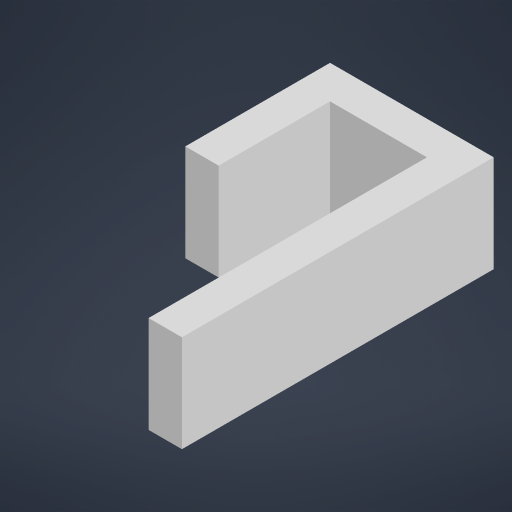
# Autodesk Inventor part: Hook_TestFit
Saved by Autodesk Inventor 2024 (Build 280153000, 153)
## iProperties
Created: 2023-07-11
Part Number: Hook_TestFit
Material: Generic
Document SubType Name: Modeling
Designer: User
Density: 1 g/cm^3
Appearance: Default
Author: User
Autodesk Inventor part; units mm, degrees
ref_plane "YZ Plane" through (0, 0, 0) normal (1, 0, 0) x (0, 1, 0)
ref_plane "XZ Plane" through (0, 0, 0) normal (0, 1, 0) x (-1, 0, 0)
ref_plane "XY Plane" through (0, 0, 0) normal (0, 0, 1) x (1, 0, 0)
sketch "Sketch1" plane through (0, 0, 0) normal (0, 0, 1) x (1, 0, 0)
  line L0 (0, 0) -> (-8.7, 0)
  line L1 (-8.7, 0) -> (-8.7, 8.7)
  line L2 (-8.7, 8.7) -> (0, 8.7)
  line L3 (0, 8.7) -> (0, 0)
  dimension "d0" = 8.7
  dimension "d1" = 8.7
  constraints: 8 end point, 2 parallel, 1 horizontal, 1 perpendicular
  measures "d0" distance of L1.end L2.end
  measures "d1" distance of L0.end L1.end
extrude "Extrusion1" add sketch "Sketch1" along normal blind 3
sketch "Sketch2" plane through (-8.7, 0, 0) normal (-1, 0, 0) x (0, 0, 1)
  line L0 (0, 8.7) -> (0, 0) projected
  line L1 (0, 0) -> (3, 0)
  line L2 (3, 0) -> (3, 8.7)
  line L3 (3, 8.7) -> (0, 8.7)
  line L4 (0, 8.7) -> (0, 0)
  constraints: 8 end point, 2 parallel, 1 horizontal, 1 perpendicular
extrude "Extrusion2" add sketch "Sketch2" along normal blind 3
sketch "Sketch3" plane through (0, 0, 3) normal (0, 0, 1) x (1, 0, 0)
  line L0 (0, 8.7) -> (-11.7, 8.7) projected
  line L1 (0, 0) -> (-11.7, 0) projected
  line L2 (-11.7, 8.7) -> (-8.7, 8.7)
  line L3 (-8.7, 8.7) -> (-8.7, 0)
  line L4 (-8.7, 0) -> (-11.7, 0)
  line L5 (-11.7, 0) -> (-11.7, 8.7)
  dimension "d6" = 3
  constraints: 8 end point, 2 parallel, 1 horizontal, 1 perpendicular, 1 point on line
  measures "d6" distance of L3.end L4.end
extrude "Extrusion3" add sketch "Sketch3" along normal blind 10
sketch "Sketch5" plane through (0, 0, 0) normal (1, 0, 0) x (0, 0, -1)
  line L0 (0, 8.7) -> (-3, 8.7) projected
  line L1 (0, 0) -> (-3, 0)
  line L2 (-3, 0) -> (-3, 8.7)
  line L3 (-3, 8.7) -> (0, 8.7)
  line L4 (0, 8.7) -> (0, 0)
  dimension "d9" = 3
  constraints: 8 end point, 2 parallel, 1 horizontal, 1 perpendicular
  measures "d9" distance of L0.end L3.end
extrude "Extrusion4" add sketch "Sketch5" along normal blind 3
sketch "Sketch6" plane through (0, 0, 3) normal (0, 0, 1) x (1, 0, 0)
  line L0 (3, 8.7) -> (-11.7, 8.7) projected
  line L1 (3, 8.7) -> (0, 8.7)
  line L2 (0, 8.7) -> (0, 0)
  line L3 (0, 0) -> (3, 0)
  line L4 (3, 0) -> (3, 8.7)
  constraints: 8 end point, 2 parallel, 1 horizontal, 1 perpendicular
extrude "Extrusion5" add sketch "Sketch6" along normal blind 25
body "Solid1"
